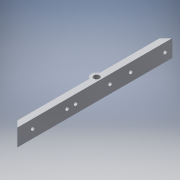
# Autodesk Inventor part: Gearbox Support Thing
Saved by Autodesk Inventor 2019.4 (Build 234330000, 330)
## iProperties
Created: 2020-01-06
Part Number: Gearbox Support Thing
Material: ABS Plastic
Document SubType Name: Modeling
Designer: Mark
Mass: 29.68 g
Surface Area: 65.4 cm^2
Volume: 28 cm^3
Density: 1.06 g/cm^3
Appearance: Smooth - White
Author: Mark
Autodesk Inventor part; units mm, degrees
ref_plane "YZ Plane" through (0, 0, 0) normal (1, 0, 0) x (0, 1, 0)
ref_plane "XZ Plane" through (0, 0, 0) normal (0, 1, 0) x (-1, 0, 0)
ref_plane "XY Plane" through (0, 0, 0) normal (0, 0, 1) x (1, 0, 0)
sketch "Sketch1" plane through (0, 0, 0) normal (1, 0, 0) x (0, 1, 0)
  line L0 (-12.5, 35) -> (12.5, 35)
  line L1 (12.5, 35) -> (12.5, -35)
  line L2 (12.5, -35) -> (-12.5, -35)
  line L3 (-12.5, -35) -> (-12.5, 35)
  line L4 (-12.5, 35) -> (12.5, -35) construction
  line L5 (12.5, 35) -> (-12.5, -35) construction
  point P0 (0, 0)
  dimension "d0" = 25
  dimension "d1" = 70
  constraints: 12 end point, 2 midpoint, 2 parallel, 1 horizontal, 1 perpendicular
  measures "d0" distance of L1.end L2.end
  measures "d1" distance of L0.end L1.end
extrude "Extrusion1" add sketch "Sketch1" along normal blind 14
sketch "Sketch2" plane through (0, 0, 0) normal (-1, 0, 0) x (0, 0, 1)
  circle A0 centre (-25, 0) radius 2.75
  circle A1 centre (25, 0) radius 2.75
  line L0 (-35, -12.5) -> (35, -12.5) projected
  line L1 (-35, 12.5) -> (-35, -12.5) projected
  point P0 (0, 0)
  dimension "d4" = 5.5
  dimension "d5" = 5.5
  dimension "d6" = 12.5
  dimension "d7" = 50
  dimension "d8" = 12.5
  dimension "d9" = 10
  constraints: 2 centre point
  measures "d4" diameter of A0
  measures "d5" diameter of A1
  measures "d6" distance from line of L0 A0.centre
  measures "d7" distance of A1.centre A0.centre
  measures "d8" distance from line of L0 A1.centre
  measures "d9" distance from line of L1 A0.centre
extrude "Extrusion2" cut sketch "Sketch2" against normal blind 16
sketch "Sketch3" plane through (0, 12.5, 35) normal (0, 1, 0) x (1, 0, 0)
  circle A0 centre (8, 46.125) radius 4.25
  line L0 (0, 70) -> (14, 70) projected
  line L1 (0, 0) -> (0, 70) projected
  circle A1 centre (8, 46.125) radius 8
  point P0 (0, 35)
  dimension "d12" = 8.5
  dimension "d13" = 23.875
  dimension "d14" = 8
  dimension "d15" = 16
  constraints: 2 centre point, 1 coincident
  measures "d12" diameter of A0
  measures "d13" distance from line of L0 A0.centre
  measures "d14" distance from line of L1 A0.centre
  measures "d15" diameter of A1
extrude "Extrusion3" cut sketch "Sketch3" against normal blind 25 contours A0
sketch "Sketch4" plane through (0, 12.5, 35) normal (0, 1, 0) x (1, 0, 0)
  circle A0 centre (8, 46.125) radius 8
  circle A1 centre (8, 46.125) radius 4.25 projected
  line L0 (5, 53.5412) -> (5, 70)
  line L1 (0, 0) -> (0, 70) projected
  line L2 (0, 0) -> (14, 0) projected
  line L3 (7.2683, 38.1585) -> (45.4268, 38.1585) construction
  line L4 (5, 38.7088) -> (5, 0)
  line L5 (5, 53.5412) -> (58.5412, 53.5412) construction
  line L6 (5, 70) -> (0, 70)
  line L7 (5, 0) -> (0, 0)
  line L8 (0, 0) -> (0, 70)
  point P0 (0, 35)
  dimension "d18" = 16
  dimension "d19" = 5
  dimension "d21" = 90
  dimension "d22" = 5
  constraints: 14 end point, 3 point on circle, 2 horizontal, 2 perpendicular, 1 centre point, 1 concentric, 1 parallel, 1 point on line, 1 vertical
  measures "d18" diameter of A0
  measures "d19" distance between parallel lines of L0 L1
  measures "d21" angle of L4 L5
  measures "d22" distance from line of point (0, 35) L4
extrude "Extrusion4" cut sketch "Sketch4" against normal blind 41.5 contours A0 L1 L6 L0 | L4 L2 L1 A0
sketch "Sketch5" plane through (5, 12.5, -35) normal (-1, 0, 0) x (0, 0, 1)
  line L0 (0, 0) -> (70, 0) projected
  line L1 (70, 0) -> (150, 0)
  line L2 (150, 0) -> (150, -25)
  line L3 (150, -25) -> (70, -25)
  line L4 (70, -25) -> (70, 0)
  line L5 (0, -25) -> (0, 0) projected
  line L6 (0, -25) -> (-10, -25)
  line L7 (-10, -25) -> (-10, 0)
  line L8 (-10, 0) -> (0, 0)
  line L9 (0, 0) -> (0, -25)
  point P0 (35, -12.5)
  dimension "d26" = 80
  dimension "d27" = 25
  dimension "d28" = 10
  dimension "d29" = 25
  constraints: 16 end point, 4 parallel, 2 horizontal, 2 perpendicular
  measures "d26" distance of L2.end L3.end
  measures "d27" distance of L1.end L2.end
  measures "d28" distance of L7.end L8.end
  measures "d29" distance of L6.end L7.end
extrude "Extrusion5" add sketch "Sketch5" against normal blind 9
chamfer "Chamfer1" distance 9 angle 45 1 edges at (5, 0, 115)
sketch "Sketch6" plane through (5, -12.5, -18.5412) normal (-1, 0, 0) x (0, 0, 1)
  circle A0 centre (70.7082, 12.5) radius 2.75
  circle A1 centre (120.7082, 12.5) radius 2.75
  line L0 (124.5412, 0) -> (14.8324, 0) projected
  line L1 (0, 0) -> (14.8324, 0) projected
  circle A2 centre (-6.4588, 12.5) radius 2.75 projected
  circle A3 centre (43.5412, 12.5) radius 2.75 projected
  point P0 (18.5412, 12.5)
  point P1 (-87.4588, 0)
  dimension "d35" = 5.5
  dimension "d36" = 5.5
  dimension "d40" = 50
  dimension "d41" = 12.5
  dimension "d42" = 12.5
  dimension "d46" = 27.167
  constraints: 2 centre point
  measures "d35" diameter of A0
  measures "d36" diameter of A1
  measures "d40" distance of A0.centre A1.centre
  measures "d41" distance from line of L0 A1.centre
  measures "d42" distance from line of L0 A0.centre
  measures "d46" distance of A3.centre A0.centre
extrude "Extrusion6" cut sketch "Sketch6" against normal blind 9
chamfer "Chamfer3" distance 9 angle 45 1 edges at (5, 0, -45)
body "Solid1"
